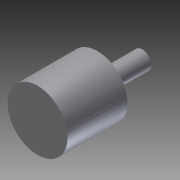
# Autodesk Inventor part: Silenbloc
Saved by Autodesk Inventor 2012 (Build 160160000, 160)
## iProperties
Created: 2013-03-13
Part Number: Silenbloc
Material: Default
Document SubType Name: Modeling
Designer: mce
Density: 1 g/cm^3
Author: mce
Autodesk Inventor part; units mm, degrees
ref_plane "YZ Plane" through (0, 0, 0) normal (1, 0, 0) x (0, 1, 0)
ref_plane "XZ Plane" through (0, 0, 0) normal (0, 1, 0) x (-1, 0, 0)
ref_plane "XY Plane" through (0, 0, 0) normal (0, 0, 1) x (1, 0, 0)
sketch "Sketch1" plane through (0, 0, 0) normal (0, 0, 1) x (1, 0, 0)
  line L0 (0, 0) -> (10, 0)
  line L1 (10, 0) -> (10, 20)
  line L2 (10, 20) -> (3, 20)
  line L3 (3, 20) -> (3, 35)
  line L4 (3, 35) -> (0, 35)
  line L5 (0, 27.6527) -> (0, -18.7044) construction
  line L6 (0, 35) -> (0, 0)
  dimension "d0" = 10
  dimension "d1" = 3
  dimension "d2" = 15
  dimension "d3" = 20
  constraints: 14 end point, 2 point on line, 1 horizontal, 1 vertical
  measures "d0" distance between parallel lines of L5 L1
  measures "d1" distance between parallel lines of L5 L3
  measures "d2" distance between parallel lines of L2 L4
  measures "d3" distance between parallel lines of L0 L2
revolve "Revolution1" add sketch "Sketch1" angle 360 about axis through (0, 27.6527, 0) along (0, -1, 0)
body "Solid1"
